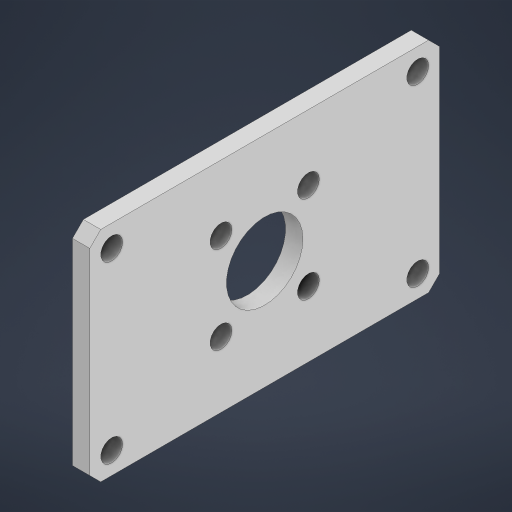
# Autodesk Inventor part: TurretMotorPlate
Saved by Autodesk Inventor 2024 (Build 280153000, 153)
## iProperties
Created: 2023-10-26
Part Number: TurretMotorPlate
Material: Generic
Document SubType Name: Modeling
Designer: avsar
Density: 1 g/cm^3
Appearance: Default
Author: avsar
Autodesk Inventor part; units mm, degrees
ref_plane "YZ Plane" through (0, 0, 0) normal (1, 0, 0) x (0, 1, 0)
ref_plane "XZ Plane" through (0, 0, 0) normal (0, 1, 0) x (-1, 0, 0)
ref_plane "XY Plane" through (0, 0, 0) normal (0, 0, 1) x (1, 0, 0)
sketch "Sketch1" plane through (0, 0, 0) normal (1, 0, 0) x (0, 1, 0)
  line L0 (-20, 32) -> (20, 32)
  line L1 (20, 32) -> (20, -32)
  line L2 (20, -32) -> (-20, -32)
  line L3 (-20, -32) -> (-20, 32)
  line L4 (-20, 32) -> (20, -32) construction
  line L5 (20, 32) -> (-20, -32) construction
  point P0 (0, 0)
  dimension "d0" = 40
  dimension "d1" = 64
  constraints: 12 end point, 2 midpoint, 2 parallel, 1 horizontal, 1 perpendicular
  measures "d0" distance of L1.end L2.end
  measures "d1" distance of L0.end L1.end
extrude "Extrusion1" add sketch "Sketch1" along normal mid plane 3.175
sketch "Sketch2" plane through (1.5875, 0, 0) normal (1, 0, 0) x (0, 0, -1)
  circle A0 centre (-28, 16) radius 2
  line L0 (-32, 20) -> (-32, -20) construction
  line L1 (-32, 0) -> (32, 0) construction
  line L2 (32, -20) -> (32, 20) construction
  line L3 (32, 20) -> (-32, 20) construction
  line L4 (0, 20) -> (0, -20) construction
  circle A1 centre (28, 16) radius 2
  circle A2 centre (-28, -16) radius 2
  circle A3 centre (28, -16) radius 2
  circle A4 centre (-8, 8) radius 2
  circle A5 centre (-8, -8) radius 2
  circle A6 centre (8, -8) radius 2
  circle A7 centre (8, 8) radius 2
  circle A8 centre (0, 0) radius 7
  point P0 (0, 0)
  point P1 (0, 0)
  dimension "d4" = 4
  dimension "d5" = 28
  dimension "d6" = 16
  dimension "d7" = 4
  dimension "d8" = 8
  dimension "d9" = 8
  dimension "d12" = 360
  dimension "d14" = 14
  constraints: 9 centre point, 5 midpoint, 4 end point, 3 symmetric about line, 1 coincident, 1 vertical, 12 other
  measures "d4" diameter of A0
  measures "d5" horizontal distance of point (0, 0) A0.centre
  measures "d6" vertical distance of point (0, 0) A0.centre
  measures "d7" diameter of A4
  measures "d8" horizontal distance of point (0, 0) A4.centre
  measures "d9" horizontal distance of point (0, 0) A4.centre
  measures "d14" diameter of A8
extrude "Extrusion2" cut sketch "Sketch2" against normal through all
chamfer "Chamfer1" distance 2 angle 45 4 edges at (0, 20, 32) (0, -20, 32) (0, -20, -32) (0, 20, -32)
body "Solid1"
